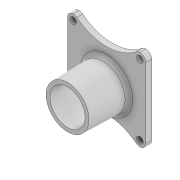
# Autodesk Inventor part: 22mm to oxymountV2
Saved by Autodesk Inventor 2020 (Build 240168000, 168)
## iProperties
Created: 2020-05-08
Part Number: 22mm to oxymountV2
Material: Generic
Document SubType Name: Modeling
Designer: rayan
Density: 1 g/cm^3
Appearance: Default
Author: rayan
Autodesk Inventor part; units mm, degrees
ref_plane "YZ Plane" through (0, 0, 0) normal (1, 0, 0) x (0, 1, 0)
ref_plane "XZ Plane" through (0, 0, 0) normal (0, 1, 0) x (-1, 0, 0)
ref_plane "XY Plane" through (0, 0, 0) normal (0, 0, 1) x (1, 0, 0)
sketch "Sketch3" plane through (0, 0, 0) normal (0, 0, 1) x (1, 0, 0)
  line L0 (-20.1, 21) -> (20.1, 21)
  line L1 (20.1, 21) -> (20.1, -21)
  line L2 (20.1, -21) -> (-20.1, -21)
  line L3 (-20.1, -21) -> (-20.1, 21)
  line L4 (-20.1, 21) -> (20.1, -21) construction
  line L5 (20.1, 21) -> (-20.1, -21) construction
  point P0 (0, 0)
  dimension "d24" = 40.2
  dimension "d25" = 42
  constraints: 12 end point, 2 midpoint, 2 parallel, 1 horizontal, 1 perpendicular
  measures "d24" distance of L1.end L2.end
  measures "d25" distance of L0.end L1.end
extrude "Extrusion3" add sketch "Sketch3" along normal blind 3
sketch "Sketch4" plane through (0, 0, 3) normal (0, 0, 1) x (1, 0, 0)
  line L0 (20.1, 21) -> (-20.1, 21) projected
  line L1 (-20.1, 21) -> (-17.1, 21) construction
  line L2 (-17.1, 21) -> (-17.1, 18) construction
  line L3 (-17.1, 18) -> (-20.1, 18) construction
  line L4 (-20.1, 18) -> (-20.1, 21) construction
  circle A0 centre (-17.1, 18) radius 1.7
  point P0 (0, 0)
  dimension "d28" = 3
  dimension "d29" = 3
  dimension "d30" = 3.4
  constraints: 8 end point, 2 parallel, 1 centre point, 1 coincident, 1 horizontal, 1 perpendicular
  measures "d28" distance of L2.end L3.end
  measures "d29" distance of L1.end L2.end
  measures "d30" diameter of A0
extrude "Extrusion4" cut sketch "Sketch4" against normal through all
fillet "Fillet2" radius 3 1 edges at (-20.1, 21, 1.5)
mirror "Mirror2" about plane through (0, 0, 0) normal (0, 1, 0) of "Fillet2", "Extrusion4"
mirror "Mirror3" about plane through (0, 0, 0) normal (1, 0, 0) of "Fillet2", "Extrusion4", "Mirror2"
sketch "Sketch5" plane through (0, 0, 3) normal (0, 0, 1) x (1, 0, 0)
  circle A0 centre (-17.1, 18) radius 1.7 construction
  circle A1 centre (17.1, 18) radius 1.7 construction
  line L0 (-17.1, 18) -> (17.1, 18) construction
  line L1 (17.1, 18) -> (17.1, 15) construction
  line L2 (17.1, 15) -> (-17.1, 15) construction
  line L3 (-17.1, 15) -> (-17.1, 18) construction
  arc A2 (-17.1, 21) -> (-20.1, 18) centre (-17.1, 18) ccw construction
  line L4 (-17.1, 18) -> (-17.1, 21) construction
  line L5 (17.1, 21) -> (-17.1, 21) construction
  line L6 (17.1, 18) -> (17.1, 21) construction
  line L7 (-17.1, 18) -> (-17.1, 21) construction
  line L8 (-17.1, 21) -> (-16, 21) construction
  line L9 (-16, 21) -> (-16, 18) construction
  line L10 (-16, 18) -> (-17.1, 18) construction
  line L11 (17.1, 18) -> (17.1, 21) construction
  line L12 (17.1, 21) -> (16, 21) construction
  line L13 (16, 21) -> (16, 18) construction
  line L14 (16, 18) -> (17.1, 18) construction
  arc A3 (-16, 21) -> (16, 21) centre (0, 39.3333) ccw
  line L15 (-16, 21) -> (16, 21)
  line L16 (17.1, 21) -> (-17.1, 21) projected
  point P0 (0, 0)
  point P1 (0, 15)
  dimension "d34" = 3
  dimension "d48" = 1.1
  dimension "d49" = 1.1
  constraints: 30 end point, 6 parallel, 3 collinear, 3 perpendicular, 3 point on circle, 2 vertical, 1 centre point, 1 horizontal, 1 midpoint
  measures "d34" distance of L0.end L1.end
  measures "d48" distance of L4.end L8.end
  measures "d49" distance between parallel lines of L13 L6
extrude "Extrusion5" cut sketch "Sketch5" against normal through all
mirror "Mirror4" about plane through (0, 0, 0) normal (0, 1, 0) of "Extrusion5"
fillet "Fillet3" radius 3 4 edges at (-16, 21, 1.5) (16, 21, 1.5) (16, -21, 1.5) (-16, -21, 1.5)
sketch "Sketch7" plane through (0, 0, 3) normal (0, 0, 1) x (1, 0, 0)
  line L0 (15.3, 7.9) -> (15.3, -11.6) construction
  line L1 (15.3, -11.6) -> (-15.4, -11.6) construction
  line L2 (-15.4, -11.6) -> (-15.4, 7.9) construction
  line L3 (-15.4, 7.9) -> (15.3, 7.9) construction
  line L4 (-17.65, -15) -> (30.6, -15) construction
  line L5 (30.6, -15) -> (30.6, 15) construction
  line L6 (30.6, 15) -> (-30.1, 15) construction
  line L7 (-30.1, 15) -> (-30.1, 10) construction
  line L8 (-17.65, 10) -> (-30.1, 10) construction
  line L9 (-17.65, 10) -> (-17.65, -15) construction
  line L10 (15.3, -11.6) -> (-15.4, 7.9) construction
  line L11 (-15.4, -11.6) -> (15.3, 7.9) construction
  line L12 (0, 0) -> (-0.05, 0) construction
  line L13 (-0.05, 0) -> (-0.05, -1.85) construction
  line L14 (-0.05, -1.85) -> (0, -1.85) construction
  line L15 (0, -1.85) -> (0, 0) construction
  circle A0 centre (0, -1.85) radius 9
  dimension "d41" = 18
  constraints: 12 end point, 2 parallel, 1 centre point, 1 coincident, 1 horizontal, 1 midpoint, 1 perpendicular
  measures "d41" diameter of A0
extrude "Extrusion6" cut sketch "Sketch7" against normal through all
sketch "Sketch8" plane through (0, 0, 3) normal (0, 0, 1) x (1, 0, 0)
  circle A0 centre (0, -1.85) radius 9 projected
  circle A1 centre (-17.1, 18) radius 1.7 projected
  circle A2 centre (-17.1, -18) radius 1.7 projected
  circle A3 centre (17.1, 18) radius 1.7 projected
  circle A4 centre (17.1, -18) radius 1.7 projected
  line L0 (20.1, -18) -> (20.1, 18) projected
  line L1 (-20.1, 18) -> (-20.1, -18) projected
  circle A5 centre (0, -1.85) radius 11
  arc A6 (17.1, -21) -> (20.1, -18) centre (17.1, -18) ccw projected
  arc A7 (20.1, 18) -> (17.1, 21) centre (17.1, 18) ccw projected
  line L2 (17.1, 21) -> (17.088, 21) projected
  arc A8 (-17.1, 21) -> (-20.1, 18) centre (-17.1, 18) ccw projected
  arc A9 (-20.1, -18) -> (-17.1, -21) centre (-17.1, -18) ccw projected
  line L3 (-17.1, -21) -> (-17.088, -21) projected
  arc A10 (15.2125, -20.3415) -> (-15.2125, -20.3415) centre (0, -39.3333) ccw projected
  line L4 (17.088, -21) -> (17.1, -21) projected
  arc A11 (-15.2125, 20.3415) -> (15.2125, 20.3415) centre (0, 39.3333) ccw projected
  line L5 (-17.088, 21) -> (-17.1, 21) projected
  arc A12 (-17.088, -21) -> (-15.2125, -20.3415) centre (-17.088, -18) ccw projected
  arc A13 (15.2125, -20.3415) -> (17.088, -21) centre (17.088, -18) ccw projected
  arc A14 (17.088, 21) -> (15.2125, 20.3415) centre (17.088, 18) ccw projected
  arc A15 (-15.2125, 20.3415) -> (-17.088, 21) centre (-17.088, 18) ccw projected
  point P0 (0, 0)
  dimension "d42" = 22
  constraints: 1 centre point, 1 coincident
  measures "d42" diameter of A5
extrude "Extrusion7" add sketch "Sketch8" along normal blind 20 contours A5
sketch "Sketch9" plane through (0, 0, 0) normal (1, 0, 0) x (0, 1, 0)
  line L0 (9.15, 23) -> (-12.85, 23) projected
  line L1 (-12.85, 3) -> (9.15, 3) projected
  line L2 (9.15, 23) -> (-12.85, 23) projected
  line L3 (9.15, 23) -> (9.15, 3) construction
  line L4 (9.15, 3) -> (9.65, 3) construction
  line L5 (9.65, 3) -> (9.65, 23) construction
  line L6 (9.65, 23) -> (9.15, 23) construction
  line L7 (-1.85, 23) -> (-1.85, 3)
  line L8 (18, 3) -> (-18, 3) projected
  line L9 (9.15, 23) -> (9.65, 3)
  line L10 (9.65, 3) -> (9.15, 3)
  line L11 (9.15, 3) -> (9.15, 23)
  point P0 (0, 0)
  point P1 (17.2722, 3)
  point P2 (-17.2722, 3)
  dimension "d45" = 0.5
  constraints: 16 end point, 4 equal length, 3 perpendicular, 1 midpoint, 1 point on line
  measures "d45" distance of L4.end L1.end
revolve "Revolution1" add sketch "Sketch9" angle 360 about axis through (0, -1.85, 23) along (0, 0, -1) contours L9 L8 L11
fillet "Fillet4" radius 2 1 edges at (0, -13.35, 3)
equation "\"d49\" = d48"
body "Solid2"
